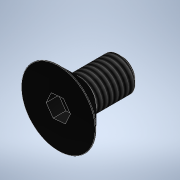
# Autodesk Inventor part: SCREW,FLAT HD,P,12.9,M8X1.25X15MM
Saved by Autodesk Inventor 2022.4 (Build 264492000, 492)
## iProperties
Manager: 100-33259
Category: _
Created: 2012-03-26
Material: Generic
Document SubType Name: Modeling
Designer: cathy.lesperance , Cathy
Description: SCREW, FLAT HD, P, 12.9, M8X1.25X15MM
Density: 1 g/cm^3
Checked By: 21MXN
Engr Approved By: P
User Status: Released
Mfg Approved By: Eric.Michaud
Appearance: Glossy - Black
Part Number: SCREW,FLAT HD,P,12.9,M8X1.25X15MM
Mass: 1.11777 g
Surface Area: 8.65901 cm^2
Volume: 1.11777 cm^3
Control State: 0
Master: False
Checked Out: False
Shininess: 64.0
Length Units: 11269
Angle Units: 11279
Time Units: 11290
Mass Units: 11283
Length Display Precision: 3
Angle Display Precision: 2
CN_SERVICEABLE: _
CN_MASS: 0.001118
CL_runCount: 1
FinishProperty: ToBeSet
FIRST_DESCRIPTION: SCREW, FLAT HD, P, 12.9, M8X1.25X15MM
SECOND_DESCRIPTION: _
THIRD_DESCRIPTION: _
CN_DETAILER: -
CN_MFG_PART_NUM: _
CN_MFG_NAME: DEFAULT
STANDARDCLASSFLAG: P
CUSTOMERNUMBER: _
CN_DESIGNER: Eric.Michaud
PTC_WM_ITERATION: 2
PTC_WM_ORGANIZATION_ID: CLWC
PTC_WM_LIFECYCLE: CLWC_CAD_LC
Density: 0.0
Volumn: 0.0
Area: 0.0
PropertySet Name: Model Information
Author: -
Subject: _
Keywords: DEFAULT
Revision Number: 1
Autodesk Inventor part; units mm, degrees
ref_plane "YZ Plane" through (0, 0, 0) normal (1, 0, 0) x (0, 1, 0)
ref_plane "XZ Plane" through (0, 0, 0) normal (0, 1, 0) x (-1, 0, 0)
ref_plane "XY Plane" through (0, 0, 0) normal (0, 0, 1) x (1, 0, 0)
sketch "Sketch1" plane through (0, 0, 0) normal (0, 0, 1) x (1, 0, 0)
  circle A0 centre (0, 0) radius 4
  dimension "Diameter" = 8
  constraints: 1 centre point
  measures "Diameter" diameter of A0
extrude "Extrusion1" add sketch "Sketch1" along normal blind 10.04
sketch "Sketch2" plane through (0, 0, 10.04) normal (0, 0, 1) x (1, 0, 0)
  circle A0 centre (0, 0) radius 4 projected
extrude "Extrusion2" add sketch "Sketch2" along normal blind 4.96 draft 45
sketch "Sketch3" plane through (0, 0, 15) normal (0, 0, 1) x (1, 0, 0)
  circle A0 centre (0, 0) radius 8.96 projected
  circle A1 centre (0, 0) radius 2.8868 construction
  line L0 (1.2084, 2.6217) -> (2.8746, 0.2644)
  line L1 (2.8746, 0.2644) -> (1.6662, -2.3573)
  line L2 (1.6662, -2.3573) -> (-1.2084, -2.6217)
  line L3 (-1.2084, -2.6217) -> (-2.8746, -0.2644)
  line L4 (-2.8746, -0.2644) -> (-1.6662, 2.3573)
  line L5 (-1.6662, 2.3573) -> (1.2084, 2.6217)
  dimension "Hex_Width" = 5
  constraints: 12 end point, 6 point on circle, 4 equal length, 1 centre point, 1 coincident
  measures "Hex_Width" distance between parallel lines of L0 L3
extrude "Extrusion3" cut sketch "Sketch3" against normal blind 3 contours L0 L1 L2 L3 L4 L5
thread "Thread1" size "M8x1.25" class "4g6g" standard "ANSI Metric M Profile" length 10.04
chamfer "Chamfer2" distance 0.8 angle 45 1 edges at (-4, 0, 0)
fillet "Fillet1" radius 0.1 1 edges at (-8.96, 0, 15)
equation "\"d10\" = Thread_Length"
equation "\"d13\" = Chamfer"
equation "\"Thread_Length\" = 10.04"
equation "\"Length\" = 15"
equation "\"Chamfer\" = 0.8"
body "Solid1"
